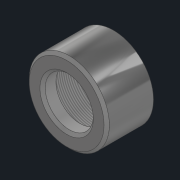
# Autodesk Inventor part: MCEN4000:B4
Saved by Autodesk Inventor 2021 (Build 250183000, 183)
## iProperties
Created: 2020-10-16
Part Number: MCEN4000:B4
Material: STAINLESS STEEL, AISI 302
Document SubType Name: Modeling
Designer: Eugene Tang
Mass: 340.563 g
Surface Area: 147.585 cm^2
Volume: 43.0711 cm^3
Density: 7.907 g/cm^3
Appearance: Rough Metal
Description: BALL SCREW DEFLECTOR FASTENER
Author: Eugene Tang
Autodesk Inventor part; units mm, degrees
ref_plane "YZ Plane" through (0, 0, 0) normal (1, 0, 0) x (0, 1, 0)
ref_plane "XZ Plane" through (0, 0, 0) normal (0, 1, 0) x (-1, 0, 0)
ref_plane "XY Plane" through (0, 0, 0) normal (0, 0, 1) x (1, 0, 0)
sketch "Sketch1" plane through (0, 0, 0) normal (0, 0, 1) x (1, 0, 0)
  circle A0 centre (0, 0) radius 23.965
  circle A1 centre (0, 0) radius 30
  spline S0 degree 3 poles (-14.0044, 16.3473) (-10.6248, 19.2425) (-6.3279, 21.0504) (-1.895, 21.4422) (2.5312, 21.8334) (7.0716, 20.8109) (10.9029, 18.5603) (14.7508, 16.3) (17.8645, 12.8114) (19.6749, 8.7325) (21.4787, 4.6683) (21.9802, 0.0378) (21.0881, -4.3184) (20.1947, -8.6815) (17.9074, -12.7482) (14.643, -15.7779) (13.057, -17.2497) (11.2477, -18.4805) (9.2962, -19.4149) knots 101.316363 101.316363 101.316363 101.316363 101.936571 101.936571 101.936571 102.555845 102.555845 102.555845 103.177798 103.177798 103.177798 103.797501 103.797501 103.797501 104.418203 104.418203 104.418203 104.719755 104.719755 104.719755 104.719755 construction
  circle A2 centre (0, 0) radius 20.7257 construction
  line L0 (9.2962, -19.4149) -> (0, 0) construction
  dimension "d0" = 47.93
  dimension "d2" = 60
  dimension "d26" = 6.035
  dimension "d27" = 21.5257
  constraints: 3 centre point, 3 coincident, 2 end point
  measures "d0" diameter of A0
  measures "d2" diameter of A1
  measures "d26" radial gap between concentric circles of A0 A1
  measures "d27" distance of L0.start L0.end
extrude "Extrusion1" add sketch "Sketch1" along normal blind 25
sketch "Sketch3" plane through (0, 0, 25) normal (0, 0, 1) x (1, 0, 0)
  circle A0 centre (0, 0) radius 23.965 construction
  circle A1 centre (0, 0) radius 30 projected
  circle A2 centre (0, 0) radius 18
  dimension "d25" = 36
  constraints: 1 centre point, 1 coincident
  measures "d25" diameter of A2
extrude "Extrusion2" add sketch "Sketch3" along normal blind 10
chamfer "Chamfer2" distance 2 angle 45 2 edges at (-30, 0, 35) (-18, 0, 35)
thread "Thread2" size "M48x1.5" class "6H" standard "ISO Metric profile" full length
equation "\"d0\" = Tread_OD"
equation "\"d2\" = NutCap_OD"
equation "\"d3\" = NutCapTread_L"
equation "\"d25\" = Screw_DIA"
equation "\"TD\" = 0.45"
equation "\"Ball_DIA\" = 6"
equation "\"Screw_L\" = 292"
equation "\"Screw_DIA\" = 36"
equation "\"Nut_OD\" = 66"
equation "\"BPath_REVQ\" = 5.75"
equation "\"Tread_OFFSET\" = 8.075"
equation "\"SteeringColumn_DIA\" = 26"
equation "\"SteeringColumnChamfer_DEG\" = 20deg"
equation "\"Rack_L\" = 307.252"
equation "\"NutCapTread_L\" = 25"
equation "\"NutCapTread_THICKNESS\" = 5.365"
equation "\"NutCap_OD\" = 60"
equation "\"SupportFlange_THICKNESS\" = 5"
equation "\"GearKey_L\" = 32"
equation "\"Tread_OD\" = 47.93"
body "Solid1"
